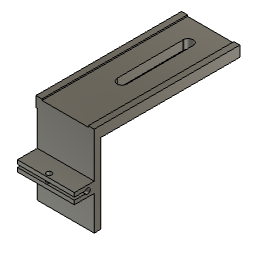
Hydrophone Mount v2 (Autodesk Fusion 360 design; units mm, degrees)
Autodesk Fusion 360 part; units mm, degrees
sketch "Sketch1" plane through (0, 0, 0) normal (0, 0, 1) x (1, 0, 0)
  line L0 (32, 42) -> (-32, 42)
  line L1 (-32, 42) -> (-32, 0)
  line L2 (-22, -68) -> (22, -68)
  line L3 (32, 0) -> (32, 42)
  line L4 (32, 42) -> (-32, -42) construction
  line L5 (-32, 42) -> (32, -42) construction
  line L6 (-32, 0) -> (-22, 0)
  line L7 (-22, 0) -> (-22, -68)
  line L8 (32, 0) -> (22, 0)
  line L9 (22, 0) -> (22, -68)
  line L10 (-3.8555, 24.984) -> (-3.6445, -25.0156)
  line L11 (3.8555, -24.984) -> (3.6445, 25.0156)
  line L12 (3.6445, 25.0156) -> (-3.6445, -25.0156) construction
  line L13 (-3.8555, 24.984) -> (3.8555, -24.984) construction
  arc A0 (3.515, 24.1268) -> (-3.7394, 24.2321) centre (-0.0988, 25.1071) ccw
  arc A1 (-3.5408, -24.3044) -> (3.7131, -24.0612) centre (0.1165, -25.0886) ccw
  line L14 (-3.8555, 24.984) -> (3.6445, 25.0156)
  line L15 (3.8555, -24.984) -> (-3.6445, -25.0156)
  line L16 (-22, 0) -> (-22, 42)
  line L17 (22, 0) -> (22, 42)
  dimension "d2" = 64
  dimension "d9" = 10
  dimension "d10" = 10
  dimension "d12" = 50
  dimension "d41" = 7.5
  dimension "d42" = 110
  constraint horizontal L0
  constraint perpendicular L0 L1
  constraint parallel L0 L2
  constraint parallel L1 L3
  constraint coincident L4 origin
  constraint coincident L5 origin
  constraint perpendicular L1 L6
  constraint perpendicular L2 L7
  constraint perpendicular L3 L8
  constraint perpendicular L2 L9
  constraint parallel L10 L11
  constraint coincident L12 origin
  constraint coincident L13 origin
  constraint coincident L11.end A0
  constraint coincident L11.start A1
  constraint coincident L13 A0.end
  constraint coincident L12 A0.start
  constraint coincident L13 A1.end
  constraint coincident L12 A1.start
  constraint perpendicular L11 L14
  constraint parallel L14 L15
  constraint coincident L0 L16.end
  constraint perpendicular L0 L16
  constraint coincident L0 L17.end
  constraint perpendicular L0 L17
  measures "d2" distance of L0.start L0.end
  measures "d9" distance of L1.end L6.end
  measures "d10" distance of L3.start L8.end
  measures "d12" distance of L10.start L10.end
  measures "d41" distance of L10 L11
  measures "d42" distance of L0 L2
extrude "Extrude2" add sketch "Sketch1" along normal blind 8 contours L0 L2 L7 L9 L16 L17
sketch "Sketch3" plane through (0, 0, 8) normal (0, 0, 1) x (-1, 0, 0)
  line L0 (-22, -42) -> (22, -42)
  line L1 (22, -42) -> (22, 68)
  line L2 (22, 68) -> (-22, 68)
  line L3 (-22, 68) -> (-22, -42)
  line L4 (-17.5, -73.8413) -> (17.5, -73.8413)
  line L5 (17.5, -73.8413) -> (17.5, 73.8413)
  line L6 (17.5, 73.8413) -> (-17.5, 73.8413)
  line L7 (-17.5, 73.8413) -> (-17.5, -73.8413)
  line L8 (-17.5, -73.8413) -> (17.5, 73.8413) construction
  line L9 (17.5, -73.8413) -> (-17.5, 73.8413) construction
  arc A0 (3.6233, 25.0155) -> (-3.8555, 24.984) centre (-0.1165, 25.0886) ccw
  line L10 (3.6233, 25.0155) -> (3.6445, 25.0156)
  line L11 (3.6445, 25.0156) -> (3.8555, -24.984)
  line L12 (3.8555, -24.984) -> (3.8411, -24.984)
  arc A1 (-3.6445, -25.0156) -> (3.8411, -24.984) centre (0.0988, -25.1071) ccw
  line L13 (-3.6445, -25.0156) -> (-3.8555, 24.984)
  dimension "d27" = 35
  constraint horizontal L4
  constraint perpendicular L4 L5
  constraint parallel L4 L6
  constraint parallel L5 L7
  constraint coincident L8 origin
  constraint coincident L9 origin
  measures "d27" distance of L4.start L4.end
extrude "Extrude3" cut sketch "Sketch3" against normal blind 1 contours L0 L2 L5 L7 | L0 L4 L5 L7 | L2 L5 L6 L7 | A0 L10 L11 L12 A1 L13
sketch "Sketch5" plane through (0, 0, 0) normal (0, 0, -1) x (1, 0, 0)
  line L0 (-22, -42) -> (22, -42)
  line L1 (22, -42) -> (22, 68)
  line L2 (22, 68) -> (-22, 68)
  line L3 (-22, 68) -> (-22, -42)
  arc A0 (3.8555, 24.984) -> (-3.6233, 25.0155) centre (0.1165, 25.0886) ccw
  line L4 (3.8555, 24.984) -> (3.6445, -25.0156)
  arc A1 (-3.8411, -24.984) -> (3.6445, -25.0156) centre (-0.0988, -25.1071) ccw
  line L5 (-3.8411, -24.984) -> (-3.8555, -24.984)
  line L6 (-3.8555, -24.984) -> (-3.6445, 25.0156)
  line L7 (-3.6445, 25.0156) -> (-3.6233, 25.0155)
  line L8 (22, 68) -> (-21, 68)
  line L9 (-21, 68) -> (-21, 63)
  line L10 (-21, 63) -> (22, 63)
  line L11 (22, 63) -> (22, 68)
  dimension "d46" = 5
  constraint horizontal L8
  constraint vertical L9
  constraint horizontal L10
  constraint vertical L11
  constraint coincident L1.end L2.start
  measures "d46" distance of L1.end L10.end
extrude "Extrude5" add sketch "Sketch5" along normal blind 60 contours L1 L2 L8 L9 L10 L11
sketch "Sketch6" plane through (0, -63, 0) normal (0, 1, 0) x (-1, 0, 0)
  line L0 (21, 0) -> (-22, 0)
  line L1 (-22, 0) -> (-22, -60)
  line L2 (-22, -60) -> (21, -60)
  line L3 (21, -60) -> (21, 0)
  line L4 (21, -30) -> (-22, -30) construction
  line L5 (0, 0) -> (0, -60) construction
  circle A0 centre (0, -45.5) radius 2.5
  circle A1 centre (0, -14.5) radius 2.5
  dimension "d59" = 5
  dimension "d60" = 5
  dimension "d61" = 15.5
  dimension "d62" = 15.5
  constraint midpoint L3 L4.start
  constraint midpoint L1 L4.end
  constraint coincident L5.start origin
  constraint coincident L2 L5.end
  constraint perpendicular L2 L5
  constraint coincident L5 A0.centre
  constraint coincident L5 A1.centre
  measures "d59" diameter of A0
  measures "d60" diameter of A1
  measures "d61" distance of L4 A1.centre
  measures "d62" distance of L4 A0.centre
sketch "Sketch7" plane through (0, -68, 0) normal (0, -1, 0) x (1, 0, 0)
  line L0 (22, -60) -> (22, 8)
  line L1 (22, 8) -> (17.5, 8)
  line L2 (17.5, 8) -> (17.5, 7)
  line L3 (17.5, 7) -> (-17.5, 7)
  line L4 (-17.5, 7) -> (-17.5, 8)
  line L5 (-17.5, 8) -> (-22, 8)
  line L6 (-22, 8) -> (-22, 0)
  line L7 (-22, 0) -> (-21, 0)
  line L8 (-21, 0) -> (-21, -60)
  line L9 (-21, -60) -> (22, -60)
  line L10 (0, 0) -> (0.5, -60)
  line L11 (0.25, -30) -> (-21, -30)
  line L12 (0.25, -30) -> (22, -30)
  line L13 (22, -32) -> (-21, -32)
  line L14 (22, -28) -> (-21, -28)
  line L15 (22, -34) -> (-21, -34)
  line L16 (-21, -26) -> (22, -26)
  dimension "d69" = 2
  dimension "d70" = 2
  dimension "d71" = 2
  dimension "d72" = 2
  constraint coincident L10.start origin
  constraint midpoint L9 L10.end
  constraint midpoint L10 L11.start
  constraint coincident L8 L11.end
  constraint perpendicular L8 L11
  constraint coincident L0 L12.end
  constraint perpendicular L0 L12
  constraint coincident L0 L13.start
  constraint coincident L8 L13.end
  constraint perpendicular L8 L13
  constraint coincident L0 L14.start
  constraint coincident L8 L14.end
  constraint perpendicular L8 L14
  constraint coincident L0 L15.start
  constraint coincident L8 L15.end
  constraint perpendicular L8 L15
  constraint coincident L8 L16.start
  constraint coincident L0 L16.end
  constraint perpendicular L0 L16
  measures "d69" distance of L12 L13
  measures "d70" distance of L12 L14
  measures "d71" distance of L13 L15
  measures "d72" distance of L14 L16
extrude "Extrude8" add sketch "Sketch7" along normal blind 10 contours L0 L10 L13 L15 | L0 L10 L12 L13 | L8 L10 L13 L15 | L0 L10 L12 L14 | L8 L10 L11 L13 | L0 L10 L14 L16 | L8 L10 L11 L14 | L8 L10 L14 L16
sketch "Sketch8" plane through (-21, 0, 0) normal (-1, 0, 0) x (0, -1, 0)
  line L0 (68, -60) -> (68, -34)
  line L1 (68, -34) -> (78, -34)
  line L2 (78, -34) -> (78, -26)
  line L3 (78, -26) -> (68, -26)
  line L4 (68, -26) -> (68, 0)
  line L5 (68, 0) -> (63, 0)
  line L6 (63, 0) -> (63, -60)
  line L7 (73, -34) -> (73, -26)
  circle A0 centre (73, -30) radius 2
  line L8 (63, -60) -> (68, -60)
  dimension "d75" = 4
  constraint midpoint L1 L7.start
  constraint midpoint L3 L7.end
  constraint midpoint L7 A0.centre
  measures "d75" diameter of A0
extrude "Extrude9" cut sketch "Sketch8" against normal blind 100 contours L7 A0 | L7 A0
sketch "Sketch9" plane through (0, -78, 0) normal (0, -1, 0) x (1, 0, 0)
  line L0 (22, -34) -> (22, -26)
  line L1 (22, -26) -> (-21, -26)
  line L2 (-21, -26) -> (-21, -34)
  line L3 (-21, -34) -> (22, -34)
  line L4 (22, -30) -> (21, -30)
  line L5 (21, -30) -> (-21, -30)
  line L6 (22, -29) -> (21, -29)
  line L7 (21, -29) -> (-21, -29)
  line L8 (22, -31) -> (21, -31)
  line L9 (21, -31) -> (-21, -31)
  dimension "d78" = 1
  dimension "d79" = -1
  constraint midpoint L0 L4.start
  constraint perpendicular L0 L4
  constraint midpoint L2 L5.end
  measures "d78" distance of L4
  measures "d79" distance of L4
extrude "Extrude10" cut sketch "Sketch9" against normal blind 5 contours L0 L2 L4 L5 L8 L9 | L0 L2 L4 L5 L6 L7
extrude "Extrude11" add 2 faces at (-6.6667, -78, -33) (-6.6667, -78, -28) along direction (0, -1, 0) blind 5
sketch "Sketch10" plane through (0, 0, -34) normal (0, 0, -1) x (1, 0, 0)
  line L0 (-21, 68) -> (22, 68)
  line L1 (22, 68) -> (22, 83)
  line L2 (22, 83) -> (-21, 83)
  line L3 (-21, 83) -> (-21, 68)
  line L4 (-21, 80) -> (22, 80)
  circle A0 centre (0, 80) radius 2
  dimension "d84" = 3
  dimension "d85" = 4
  constraint coincident L3 L4.start
  constraint coincident L1 L4.end
  constraint perpendicular L1 L4
  constraint coincident L4 A0.centre
  measures "d84" distance of L2 L4
  measures "d85" diameter of A0
extrude "Extrude12" cut sketch "Sketch10" against normal blind 100 contours L4 A0 | L4 A0
